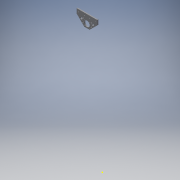
# Autodesk Inventor part: Rear Z Motor Mount
Saved by Autodesk Inventor 2017 (Build 210142000, 142)
## iProperties
Created: 2016-07-25
Part Number: Rear Z Motor Mount
Material: Generic
Document SubType Name: Modeling
Designer: User
Density: 1 g/cm^3
Appearance: Default
Author: User
Autodesk Inventor part; units mm, degrees
ref_plane "YZ Plane" through (0, 0, 0) normal (1, 0, 0) x (0, 1, 0)
ref_plane "XZ Plane" through (0, 0, 0) normal (0, 1, 0) x (-1, 0, 0)
ref_plane "XY Plane" through (0, 0, 0) normal (0, 0, 1) x (1, 0, 0)
sketch "Sketch1" plane through (0, 0, 0) normal (0, 1, 0) x (-1, 0, 0)
  line L0 (139.3953, 734.0843) -> (139.1453, 734.7093)
  line L1 (139.1453, 734.7093) -> (138.7453, 735.2093)
  line L2 (138.7453, 735.2093) -> (138.2203, 735.6093)
  line L3 (138.2203, 735.6093) -> (137.6203, 735.8593)
  line L4 (137.6203, 735.8593) -> (136.9703, 735.9593)
  line L5 (136.9703, 735.9593) -> (136.3203, 735.8593)
  line L6 (136.3203, 735.8593) -> (135.7203, 735.6093)
  line L7 (135.7203, 735.6093) -> (135.1953, 735.2093)
  line L8 (135.1953, 735.2093) -> (134.7953, 734.7093)
  line L9 (134.7953, 734.7093) -> (134.5453, 734.0843)
  line L10 (134.5453, 734.0843) -> (134.4703, 733.4343)
  line L11 (134.4703, 733.4343) -> (134.5454, 732.7843)
  line L12 (134.5454, 732.7843) -> (134.7954, 732.1844)
  line L13 (134.7954, 732.1844) -> (135.1954, 731.6593)
  line L14 (135.1954, 731.6593) -> (135.7204, 731.2593)
  line L15 (135.7204, 731.2593) -> (136.3203, 731.0093)
  line L16 (136.3203, 731.0093) -> (136.9704, 730.9343)
  line L17 (136.9704, 730.9343) -> (137.6204, 731.0094)
  line L18 (137.6204, 731.0094) -> (138.2204, 731.2594)
  line L19 (138.2204, 731.2594) -> (138.7453, 731.6593)
  line L20 (138.7453, 731.6593) -> (139.1453, 732.1843)
  line L21 (139.1453, 732.1843) -> (139.3953, 732.7843)
  line L22 (139.3953, 732.7843) -> (139.4953, 733.4341)
  line L23 (139.4953, 733.4341) -> (139.3953, 734.0843)
  line L24 (109.1446, 718.8093) -> (109.146, 712.6093)
  line L25 (109.146, 712.6093) -> (115.546, 712.6107)
  line L26 (115.546, 712.6107) -> (115.5446, 718.8107)
  line L27 (115.5446, 718.8107) -> (109.1446, 718.8093)
  line L28 (105.1702, 713.5342) -> (105.0202, 713.9092)
  line L29 (105.0202, 713.9092) -> (104.7703, 714.2342)
  line L30 (104.7703, 714.2342) -> (104.4453, 714.4842)
  line L31 (104.4453, 714.4842) -> (104.0453, 714.6593)
  line L32 (104.0453, 714.6593) -> (103.6453, 714.7093)
  line L33 (103.6453, 714.7093) -> (103.2453, 714.6593)
  line L34 (103.2453, 714.6593) -> (102.8453, 714.4842)
  line L35 (102.8453, 714.4842) -> (102.5203, 714.2343)
  line L36 (102.5203, 714.2343) -> (102.2703, 713.9093)
  line L37 (102.2703, 713.9093) -> (102.1203, 713.5343)
  line L38 (102.1203, 713.5343) -> (102.0703, 713.1093)
  line L39 (102.0703, 713.1093) -> (102.1203, 712.7093)
  line L40 (102.1203, 712.7093) -> (102.2703, 712.3093)
  line L41 (102.2703, 712.3093) -> (102.5203, 711.9843)
  line L42 (102.5203, 711.9843) -> (102.8452, 711.7343)
  line L43 (102.8452, 711.7343) -> (103.2452, 711.5841)
  line L44 (103.2452, 711.5841) -> (103.6452, 711.5341)
  line L45 (103.6452, 711.5341) -> (104.0452, 711.5841)
  line L46 (104.0452, 711.5841) -> (104.4452, 711.7341)
  line L47 (104.4452, 711.7341) -> (104.7702, 711.9841)
  line L48 (104.7702, 711.9841) -> (105.0202, 712.3091)
  line L49 (105.0202, 712.3091) -> (105.1704, 712.709)
  line L50 (105.1704, 712.709) -> (105.2452, 713.1084)
  line L51 (105.2452, 713.1084) -> (105.1702, 713.5342)
  line L52 (103.5953, 701.7594) -> (101.9953, 705.6094)
  line L53 (101.9953, 705.6094) -> (99.4703, 708.9344)
  line L54 (99.4703, 708.9344) -> (96.1453, 711.4844)
  line L55 (96.1453, 711.4844) -> (92.2953, 713.0594)
  line L56 (92.2953, 713.0594) -> (88.1453, 713.6093)
  line L57 (88.1453, 713.6093) -> (83.9953, 713.0593)
  line L58 (83.9953, 713.0593) -> (80.1453, 711.4843)
  line L59 (80.1453, 711.4843) -> (76.8203, 708.9343)
  line L60 (76.8203, 708.9343) -> (74.2953, 705.6093)
  line L61 (74.2953, 705.6093) -> (72.6953, 701.7593)
  line L62 (72.6953, 701.7593) -> (72.1453, 697.6093)
  line L63 (72.1453, 697.6093) -> (72.6953, 693.4843)
  line L64 (72.6953, 693.4843) -> (74.2953, 689.6093)
  line L65 (74.2953, 689.6093) -> (76.8203, 686.3093)
  line L66 (76.8203, 686.3093) -> (80.1453, 683.7593)
  line L67 (80.1453, 683.7593) -> (83.9953, 682.1593)
  line L68 (83.9953, 682.1593) -> (88.1453, 681.6093)
  line L69 (88.1453, 681.6093) -> (92.2953, 682.1593)
  line L70 (92.2953, 682.1593) -> (96.1453, 683.7593)
  line L71 (96.1453, 683.7593) -> (99.4703, 686.3093)
  line L72 (99.4703, 686.3093) -> (101.9953, 689.6093)
  line L73 (101.9953, 689.6093) -> (103.5953, 693.4843)
  line L74 (103.5953, 693.4843) -> (104.1453, 697.6092)
  line L75 (104.1453, 697.6092) -> (103.5953, 701.7594)
  line L76 (113.8952, 705.5088) -> (113.7453, 705.8839)
  line L77 (113.7453, 705.8839) -> (113.5201, 706.2093)
  line L78 (113.5201, 706.2093) -> (113.1952, 706.4594)
  line L79 (113.1952, 706.4594) -> (112.8451, 706.6343)
  line L80 (112.8451, 706.6343) -> (112.4451, 706.7093)
  line L81 (112.4451, 706.7093) -> (112.0451, 706.6843)
  line L82 (112.0451, 706.6843) -> (111.6701, 706.5593)
  line L83 (111.6701, 706.5593) -> (111.3201, 706.3594)
  line L84 (111.3201, 706.3594) -> (111.0451, 706.0594)
  line L85 (111.0451, 706.0594) -> (110.8702, 705.7093)
  line L86 (110.8702, 705.7093) -> (110.7703, 705.3093)
  line L87 (110.7703, 705.3093) -> (110.7703, 704.9093)
  line L88 (110.7703, 704.9093) -> (110.8704, 704.5343)
  line L89 (110.8704, 704.5343) -> (111.0454, 704.1843)
  line L90 (111.0454, 704.1843) -> (111.3203, 703.8843)
  line L91 (111.3203, 703.8843) -> (111.6703, 703.6592)
  line L92 (111.6703, 703.6592) -> (112.0453, 703.5342)
  line L93 (112.0453, 703.5342) -> (112.4453, 703.5091)
  line L94 (112.4453, 703.5091) -> (112.8453, 703.5841)
  line L95 (112.8453, 703.5841) -> (113.1954, 703.759)
  line L96 (113.1954, 703.759) -> (113.5203, 704.009)
  line L97 (113.5203, 704.009) -> (113.7452, 704.3338)
  line L98 (113.7452, 704.3338) -> (113.8952, 704.7088)
  line L99 (113.8952, 704.7088) -> (113.9453, 705.1088)
  line L100 (113.9453, 705.1088) -> (113.8952, 705.5088)
  line L101 (109.1446, 697.6093) -> (109.146, 691.4093)
  line L102 (109.146, 691.4093) -> (115.546, 691.4107)
  line L103 (115.546, 691.4107) -> (115.5446, 697.6107)
  line L104 (115.5446, 697.6107) -> (109.1446, 697.6093)
  line L105 (105.1678, 682.534) -> (105.0178, 682.909)
  line L106 (105.0178, 682.909) -> (104.7679, 683.234)
  line L107 (104.7679, 683.234) -> (104.4429, 683.484)
  line L108 (104.4429, 683.484) -> (104.0429, 683.6591)
  line L109 (104.0429, 683.6591) -> (103.6428, 683.7091)
  line L110 (103.6428, 683.7091) -> (103.2428, 683.6591)
  line L111 (103.2428, 683.6591) -> (102.8429, 683.4841)
  line L112 (102.8429, 683.4841) -> (102.5178, 683.2341)
  line L113 (102.5178, 683.2341) -> (102.2678, 682.9091)
  line L114 (102.2678, 682.9091) -> (102.1178, 682.5342)
  line L115 (102.1178, 682.5342) -> (102.0427, 682.1087)
  line L116 (102.0427, 682.1087) -> (102.1177, 681.7088)
  line L117 (102.1177, 681.7088) -> (102.2676, 681.3088)
  line L118 (102.2676, 681.3088) -> (102.5176, 680.9838)
  line L119 (102.5176, 680.9838) -> (102.8426, 680.7337)
  line L120 (102.8426, 680.7337) -> (103.2426, 680.5836)
  line L121 (103.2426, 680.5836) -> (103.6425, 680.5336)
  line L122 (103.6425, 680.5336) -> (104.0426, 680.5836)
  line L123 (104.0426, 680.5836) -> (104.4425, 680.7336)
  line L124 (104.4425, 680.7336) -> (104.7676, 680.9836)
  line L125 (104.7676, 680.9836) -> (105.0176, 681.3086)
  line L126 (105.0176, 681.3086) -> (105.1678, 681.7085)
  line L127 (105.1678, 681.7085) -> (105.2428, 682.1086)
  line L128 (105.2428, 682.1086) -> (105.1678, 682.534)
  line L129 (74.171, 682.5344) -> (74.021, 682.9094)
  line L130 (74.021, 682.9094) -> (73.7711, 683.2344)
  line L131 (73.7711, 683.2344) -> (73.4461, 683.4845)
  line L132 (73.4461, 683.4845) -> (73.0461, 683.6595)
  line L133 (73.0461, 683.6595) -> (72.6461, 683.7096)
  line L134 (72.6461, 683.7096) -> (72.2461, 683.6595)
  line L135 (72.2461, 683.6595) -> (71.8461, 683.4845)
  line L136 (71.8461, 683.4845) -> (71.5211, 683.2345)
  line L137 (71.5211, 683.2345) -> (71.2711, 682.9096)
  line L138 (71.2711, 682.9096) -> (71.1211, 682.5346)
  line L139 (71.1211, 682.5346) -> (71.0461, 682.1095)
  line L140 (71.0461, 682.1095) -> (71.121, 681.7094)
  line L141 (71.121, 681.7094) -> (71.271, 681.3095)
  line L142 (71.271, 681.3095) -> (71.521, 680.9844)
  line L143 (71.521, 680.9844) -> (71.846, 680.7344)
  line L144 (71.846, 680.7344) -> (72.2459, 680.5842)
  line L145 (72.2459, 680.5842) -> (72.6459, 680.5342)
  line L146 (72.6459, 680.5342) -> (73.0458, 680.5842)
  line L147 (73.0458, 680.5842) -> (73.4459, 680.7342)
  line L148 (73.4459, 680.7342) -> (73.7709, 680.9842)
  line L149 (73.7709, 680.9842) -> (74.0209, 681.3092)
  line L150 (74.0209, 681.3092) -> (74.1711, 681.7091)
  line L151 (74.1711, 681.7091) -> (74.246, 682.1089)
  line L152 (74.246, 682.1089) -> (74.171, 682.5344)
  line L153 (60.7446, 697.6093) -> (60.746, 691.4093)
  line L154 (60.746, 691.4093) -> (67.1456, 691.4107)
  line L155 (67.1456, 691.4107) -> (67.1442, 697.6107)
  line L156 (67.1442, 697.6107) -> (60.7446, 697.6093)
  line L157 (65.4452, 705.7089) -> (65.2453, 706.059)
  line L158 (65.2453, 706.059) -> (64.9703, 706.359)
  line L159 (64.9703, 706.359) -> (64.6204, 706.559)
  line L160 (64.6204, 706.559) -> (64.2454, 706.6841)
  line L161 (64.2454, 706.6841) -> (63.8454, 706.7092)
  line L162 (63.8454, 706.7092) -> (63.4453, 706.6342)
  line L163 (63.4453, 706.6342) -> (63.0953, 706.4592)
  line L164 (63.0953, 706.4592) -> (62.7703, 706.2093)
  line L165 (62.7703, 706.2093) -> (62.5453, 705.8843)
  line L166 (62.5453, 705.8843) -> (62.3953, 705.5093)
  line L167 (62.3953, 705.5093) -> (62.3453, 705.1093)
  line L168 (62.3453, 705.1093) -> (62.3953, 704.7093)
  line L169 (62.3953, 704.7093) -> (62.5453, 704.3343)
  line L170 (62.5453, 704.3343) -> (62.7702, 704.0093)
  line L171 (62.7702, 704.0093) -> (63.0952, 703.7592)
  line L172 (63.0952, 703.7592) -> (63.4452, 703.5842)
  line L173 (63.4452, 703.5842) -> (63.8452, 703.5092)
  line L174 (63.8452, 703.5092) -> (64.2452, 703.5342)
  line L175 (64.2452, 703.5342) -> (64.6202, 703.6591)
  line L176 (64.6202, 703.6591) -> (64.9702, 703.8841)
  line L177 (64.9702, 703.8841) -> (65.2452, 704.1841)
  line L178 (65.2452, 704.1841) -> (65.4452, 704.5341)
  line L179 (65.4452, 704.5341) -> (65.5452, 704.9091)
  line L180 (65.5452, 704.9091) -> (65.5452, 705.3089)
  line L181 (65.5452, 705.3089) -> (65.4452, 705.7089)
  line L182 (60.7203, 711.3594) -> (60.1203, 712.8093)
  line L183 (60.1203, 712.8093) -> (59.1703, 714.0343)
  line L184 (59.1703, 714.0343) -> (57.9203, 714.9843)
  line L185 (57.9203, 714.9843) -> (56.4703, 715.5843)
  line L186 (56.4703, 715.5843) -> (54.9203, 715.8093)
  line L187 (54.9203, 715.8093) -> (53.3703, 715.5843)
  line L188 (53.3703, 715.5843) -> (51.9203, 714.9843)
  line L189 (51.9203, 714.9843) -> (50.6953, 714.0343)
  line L190 (50.6953, 714.0343) -> (49.7203, 712.8093)
  line L191 (49.7203, 712.8093) -> (49.1203, 711.3593)
  line L192 (49.1203, 711.3593) -> (48.9203, 709.8093)
  line L193 (48.9203, 709.8093) -> (49.1203, 708.2343)
  line L194 (49.1203, 708.2343) -> (49.7203, 706.8093)
  line L195 (49.7203, 706.8093) -> (50.6953, 705.5593)
  line L196 (50.6953, 705.5593) -> (51.9203, 704.6093)
  line L197 (51.9203, 704.6093) -> (53.3703, 704.0093)
  line L198 (53.3703, 704.0093) -> (54.9203, 703.8093)
  line L199 (54.9203, 703.8093) -> (56.4703, 704.0093)
  line L200 (56.4703, 704.0093) -> (57.9202, 704.6093)
  line L201 (57.9202, 704.6093) -> (59.1702, 705.5594)
  line L202 (59.1702, 705.5594) -> (60.1202, 706.8094)
  line L203 (60.1202, 706.8094) -> (60.7201, 708.2344)
  line L204 (60.7201, 708.2344) -> (60.9203, 709.8095)
  line L205 (60.9203, 709.8095) -> (60.7203, 711.3594)
  line L206 (60.7446, 718.8093) -> (60.746, 712.6093)
  line L207 (60.746, 712.6093) -> (67.146, 712.6107)
  line L208 (67.146, 712.6107) -> (67.1446, 718.8107)
  line L209 (67.1446, 718.8107) -> (60.7446, 718.8093)
  line L210 (74.1702, 713.5342) -> (74.0203, 713.9092)
  line L211 (74.0203, 713.9092) -> (73.7703, 714.2342)
  line L212 (73.7703, 714.2342) -> (73.4453, 714.4842)
  line L213 (73.4453, 714.4842) -> (73.0453, 714.6593)
  line L214 (73.0453, 714.6593) -> (72.6454, 714.7093)
  line L215 (72.6454, 714.7093) -> (72.2454, 714.6593)
  line L216 (72.2454, 714.6593) -> (71.8454, 714.4843)
  line L217 (71.8454, 714.4843) -> (71.5204, 714.2343)
  line L218 (71.5204, 714.2343) -> (71.2703, 713.9093)
  line L219 (71.2703, 713.9093) -> (71.1203, 713.5343)
  line L220 (71.1203, 713.5343) -> (71.0703, 713.1093)
  line L221 (71.0703, 713.1093) -> (71.1203, 712.7093)
  line L222 (71.1203, 712.7093) -> (71.2703, 712.3093)
  line L223 (71.2703, 712.3093) -> (71.5203, 711.9843)
  line L224 (71.5203, 711.9843) -> (71.8452, 711.7342)
  line L225 (71.8452, 711.7342) -> (72.2452, 711.5841)
  line L226 (72.2452, 711.5841) -> (72.6452, 711.5341)
  line L227 (72.6452, 711.5341) -> (73.0452, 711.5841)
  line L228 (73.0452, 711.5841) -> (73.4452, 711.7341)
  line L229 (73.4452, 711.7341) -> (73.7702, 711.9841)
  line L230 (73.7702, 711.9841) -> (74.0203, 712.3091)
  line L231 (74.0203, 712.3091) -> (74.1704, 712.709)
  line L232 (74.1704, 712.709) -> (74.2453, 713.1084)
  line L233 (74.2453, 713.1084) -> (74.1702, 713.5342)
  line L234 (76.5953, 734.0843) -> (76.3453, 734.7093)
  line L235 (76.3453, 734.7093) -> (75.9453, 735.2093)
  line L236 (75.9453, 735.2093) -> (75.4203, 735.6093)
  line L237 (75.4203, 735.6093) -> (74.8203, 735.8593)
  line L238 (74.8203, 735.8593) -> (74.1703, 735.9593)
  line L239 (74.1703, 735.9593) -> (73.5203, 735.8593)
  line L240 (73.5203, 735.8593) -> (72.9203, 735.6093)
  line L241 (72.9203, 735.6093) -> (72.3953, 735.2093)
  line L242 (72.3953, 735.2093) -> (71.9953, 734.7093)
  line L243 (71.9953, 734.7093) -> (71.7453, 734.0843)
  line L244 (71.7453, 734.0843) -> (71.6703, 733.4343)
  line L245 (71.6703, 733.4343) -> (71.7453, 732.7843)
  line L246 (71.7453, 732.7843) -> (71.9954, 732.1843)
  line L247 (71.9954, 732.1843) -> (72.3953, 731.6593)
  line L248 (72.3953, 731.6593) -> (72.9203, 731.2593)
  line L249 (72.9203, 731.2593) -> (73.5203, 731.0093)
  line L250 (73.5203, 731.0093) -> (74.1704, 730.9343)
  line L251 (74.1704, 730.9343) -> (74.8203, 731.0094)
  line L252 (74.8203, 731.0094) -> (75.4203, 731.2594)
  line L253 (75.4203, 731.2594) -> (75.9453, 731.6593)
  line L254 (75.9453, 731.6593) -> (76.3453, 732.1844)
  line L255 (76.3453, 732.1844) -> (76.5953, 732.7843)
  line L256 (76.5953, 732.7843) -> (76.6953, 733.4342)
  line L257 (76.6953, 733.4342) -> (76.5953, 734.0843)
  line L258 (104.5702, 734.0842) -> (104.3202, 734.7093)
  line L259 (104.3202, 734.7093) -> (103.9202, 735.2092)
  line L260 (103.9202, 735.2092) -> (103.3952, 735.6092)
  line L261 (103.3952, 735.6092) -> (102.7703, 735.8592)
  line L262 (102.7703, 735.8592) -> (102.1203, 735.9592)
  line L263 (102.1203, 735.9592) -> (101.4702, 735.8592)
  line L264 (101.4702, 735.8592) -> (100.8452, 735.6093)
  line L265 (100.8452, 735.6093) -> (100.3202, 735.2093)
  line L266 (100.3202, 735.2093) -> (99.9202, 734.7093)
  line L267 (99.9202, 734.7093) -> (99.6702, 734.0843)
  line L268 (99.6702, 734.0843) -> (99.5702, 733.4343)
  line L269 (99.5702, 733.4343) -> (99.6702, 732.7843)
  line L270 (99.6702, 732.7843) -> (99.9202, 732.1843)
  line L271 (99.9202, 732.1843) -> (100.3202, 731.6593)
  line L272 (100.3202, 731.6593) -> (100.8452, 731.2593)
  line L273 (100.8452, 731.2593) -> (101.4702, 731.0093)
  line L274 (101.4702, 731.0093) -> (102.1202, 730.9343)
  line L275 (102.1202, 730.9343) -> (102.7702, 731.0093)
  line L276 (102.7702, 731.0093) -> (103.3952, 731.2593)
  line L277 (103.3952, 731.2593) -> (103.9201, 731.6592)
  line L278 (103.9201, 731.6592) -> (104.3201, 732.1842)
  line L279 (104.3201, 732.1842) -> (104.5701, 732.7841)
  line L280 (104.5701, 732.7841) -> (104.6702, 733.4343)
  line L281 (104.6702, 733.4343) -> (104.5702, 734.0842)
  line L282 (41.7452, 734.0843) -> (41.4953, 734.7094)
  line L283 (41.4953, 734.7094) -> (41.0953, 735.2093)
  line L284 (41.0953, 735.2093) -> (40.5703, 735.6093)
  line L285 (40.5703, 735.6093) -> (39.9703, 735.8593)
  line L286 (39.9703, 735.8593) -> (39.3203, 735.9593)
  line L287 (39.3203, 735.9593) -> (38.6703, 735.8593)
  line L288 (38.6703, 735.8593) -> (38.0703, 735.6093)
  line L289 (38.0703, 735.6093) -> (37.5453, 735.2093)
  line L290 (37.5453, 735.2093) -> (37.1453, 734.7093)
  line L291 (37.1453, 734.7093) -> (36.8953, 734.0843)
  line L292 (36.8953, 734.0843) -> (36.7953, 733.4343)
  line L293 (36.7953, 733.4343) -> (36.8953, 732.7843)
  line L294 (36.8953, 732.7843) -> (37.1453, 732.1843)
  line L295 (37.1453, 732.1843) -> (37.5453, 731.6593)
  line L296 (37.5453, 731.6593) -> (38.0703, 731.2593)
  line L297 (38.0703, 731.2593) -> (38.6703, 731.0093)
  line L298 (38.6703, 731.0093) -> (39.3203, 730.9343)
  line L299 (39.3203, 730.9343) -> (39.9703, 731.0094)
  line L300 (39.9703, 731.0094) -> (40.5703, 731.2594)
  line L301 (40.5703, 731.2594) -> (41.0953, 731.6594)
  line L302 (41.0953, 731.6594) -> (41.4953, 732.1844)
  line L303 (41.4953, 732.1844) -> (41.7453, 732.7844)
  line L304 (41.7453, 732.7844) -> (41.8203, 733.4343)
  line L305 (41.8203, 733.4343) -> (41.7452, 734.0843)
  line L306 (29.3173, 745.6342) -> (29.3233, 718.4343)
  line L307 (29.3233, 718.4343) -> (72.6578, 675.1188)
  line L308 (72.6578, 675.1188) -> (103.6578, 675.1256)
  line L309 (103.6578, 675.1256) -> (146.9733, 718.4601)
  line L310 (146.9733, 718.4601) -> (146.9673, 745.66)
  line L311 (146.9673, 745.66) -> (29.3173, 745.6342)
  line L312 (127.1703, 711.3593) -> (126.5703, 712.8093)
  line L313 (126.5703, 712.8093) -> (125.5952, 714.0343)
  line L314 (125.5952, 714.0343) -> (124.3702, 714.9843)
  line L315 (124.3702, 714.9843) -> (122.9202, 715.5843)
  line L316 (122.9202, 715.5843) -> (121.3702, 715.8093)
  line L317 (121.3702, 715.8093) -> (119.8202, 715.5843)
  line L318 (119.8202, 715.5843) -> (118.3703, 714.9843)
  line L319 (118.3703, 714.9843) -> (117.1203, 714.0342)
  line L320 (117.1203, 714.0342) -> (116.1703, 712.8092)
  line L321 (116.1703, 712.8092) -> (115.5703, 711.3592)
  line L322 (115.5703, 711.3592) -> (115.3703, 709.8092)
  line L323 (115.3703, 709.8092) -> (115.5703, 708.2342)
  line L324 (115.5703, 708.2342) -> (116.1703, 706.8092)
  line L325 (116.1703, 706.8092) -> (117.1204, 705.5592)
  line L326 (117.1204, 705.5592) -> (118.3704, 704.6093)
  line L327 (118.3704, 704.6093) -> (119.8204, 704.0093)
  line L328 (119.8204, 704.0093) -> (121.3704, 703.8093)
  line L329 (121.3704, 703.8093) -> (122.9204, 704.0093)
  line L330 (122.9204, 704.0093) -> (124.3704, 704.6093)
  line L331 (124.3704, 704.6093) -> (125.5954, 705.5593)
  line L332 (125.5954, 705.5593) -> (126.5701, 706.8093)
  line L333 (126.5701, 706.8093) -> (127.1701, 708.2343)
  line L334 (127.1701, 708.2343) -> (127.3703, 709.8093)
  line L335 (127.3703, 709.8093) -> (127.1703, 711.3593)
  point P0 (0, 0)
  constraints: 672 end point, 122 parallel, 97 perpendicular
extrude "Extrusion1" add sketch "Sketch1" along normal blind 6 contours L281 L280 L279 L278 L277 L276 L275 L274 L273 L272 L271 L270 L269 L268 L267 L266 L265 L264 L263 L262 L261 L260 L259 L258 | L311 L310 L309 L308 L307 L306
sketch "Sketch2" plane through (0, 0, 0) normal (0, -1, 0) x (1, 0, 0)
  line L0 (-104.1453, 697.6092) -> (-103.5953, 701.7594) projected
  line L1 (-103.5953, 701.7594) -> (-101.9953, 705.6094) projected
  line L2 (-101.9953, 705.6094) -> (-99.4703, 708.9344) projected
  line L3 (-99.4703, 708.9344) -> (-96.1453, 711.4844) projected
  line L4 (-96.1453, 711.4844) -> (-92.2953, 713.0594) projected
  line L5 (-92.2953, 713.0594) -> (-88.1453, 713.6093) projected
  line L6 (-88.1453, 713.6093) -> (-83.9953, 713.0593) projected
  line L7 (-83.9953, 713.0593) -> (-80.1453, 711.4843) projected
  line L8 (-80.1453, 711.4843) -> (-76.8203, 708.9343) projected
  line L9 (-76.8203, 708.9343) -> (-74.2953, 705.6093) projected
  line L10 (-74.2953, 705.6093) -> (-72.6953, 701.7593) projected
  line L11 (-72.6953, 701.7593) -> (-72.1453, 697.6093) projected
  line L12 (-72.1453, 697.6093) -> (-72.6953, 693.4843) projected
  line L13 (-72.6953, 693.4843) -> (-74.2953, 689.6093) projected
  line L14 (-74.2953, 689.6093) -> (-76.8203, 686.3093) projected
  line L15 (-76.8203, 686.3093) -> (-80.1453, 683.7593) projected
  line L16 (-80.1453, 683.7593) -> (-83.9953, 682.1593) projected
  line L17 (-83.9953, 682.1593) -> (-88.1453, 681.6093) projected
  line L18 (-88.1453, 681.6093) -> (-92.2953, 682.1593) projected
  line L19 (-92.2953, 682.1593) -> (-96.1453, 683.7593) projected
  line L20 (-96.1453, 683.7593) -> (-99.4703, 686.3093) projected
  line L21 (-99.4703, 686.3093) -> (-101.9953, 689.6093) projected
  line L22 (-101.9953, 689.6093) -> (-103.5953, 693.4843) projected
  line L23 (-103.5953, 693.4843) -> (-104.1453, 697.6092) projected
  line L24 (-127.3703, 709.8093) -> (-127.1703, 711.3593) projected
  line L25 (-127.1703, 711.3593) -> (-126.5703, 712.8093) projected
  line L26 (-126.5703, 712.8093) -> (-125.5952, 714.0343) projected
  line L27 (-125.5952, 714.0343) -> (-124.3702, 714.9843) projected
  line L28 (-124.3702, 714.9843) -> (-122.9202, 715.5843) projected
  line L29 (-122.9202, 715.5843) -> (-121.3702, 715.8093) projected
  line L30 (-121.3702, 715.8093) -> (-119.8202, 715.5843) projected
  line L31 (-119.8202, 715.5843) -> (-118.3703, 714.9843) projected
  line L32 (-118.3703, 714.9843) -> (-117.1203, 714.0342) projected
  line L33 (-117.1203, 714.0342) -> (-116.1703, 712.8092) projected
  line L34 (-116.1703, 712.8092) -> (-115.5703, 711.3592) projected
  line L35 (-115.5703, 711.3592) -> (-115.3703, 709.8092) projected
  line L36 (-115.3703, 709.8092) -> (-115.5703, 708.2342) projected
  line L37 (-115.5703, 708.2342) -> (-116.1703, 706.8092) projected
  line L38 (-116.1703, 706.8092) -> (-117.1204, 705.5592) projected
  line L39 (-117.1204, 705.5592) -> (-118.3704, 704.6093) projected
  line L40 (-118.3704, 704.6093) -> (-119.8204, 704.0093) projected
  line L41 (-119.8204, 704.0093) -> (-121.3704, 703.8093) projected
  line L42 (-121.3704, 703.8093) -> (-122.9204, 704.0093) projected
  line L43 (-122.9204, 704.0093) -> (-124.3704, 704.6093) projected
  line L44 (-124.3704, 704.6093) -> (-125.5954, 705.5593) projected
  line L45 (-125.5954, 705.5593) -> (-126.5701, 706.8093) projected
  line L46 (-126.5701, 706.8093) -> (-127.1701, 708.2343) projected
  line L47 (-127.1701, 708.2343) -> (-127.3703, 709.8093) projected
  line L48 (-60.9203, 709.8095) -> (-60.7203, 711.3594) projected
  line L49 (-60.7203, 711.3594) -> (-60.1203, 712.8093) projected
  line L50 (-60.1203, 712.8093) -> (-59.1703, 714.0343) projected
  line L51 (-59.1703, 714.0343) -> (-57.9203, 714.9843) projected
  line L52 (-57.9203, 714.9843) -> (-56.4703, 715.5843) projected
  line L53 (-56.4703, 715.5843) -> (-54.9203, 715.8093) projected
  line L54 (-54.9203, 715.8093) -> (-53.3703, 715.5843) projected
  line L55 (-53.3703, 715.5843) -> (-51.9203, 714.9843) projected
  line L56 (-51.9203, 714.9843) -> (-50.6953, 714.0343) projected
  line L57 (-50.6953, 714.0343) -> (-49.7203, 712.8093) projected
  line L58 (-49.7203, 712.8093) -> (-49.1203, 711.3593) projected
  line L59 (-49.1203, 711.3593) -> (-48.9203, 709.8093) projected
  line L60 (-48.9203, 709.8093) -> (-49.1203, 708.2343) projected
  line L61 (-49.1203, 708.2343) -> (-49.7203, 706.8093) projected
  line L62 (-49.7203, 706.8093) -> (-50.6953, 705.5593) projected
  line L63 (-50.6953, 705.5593) -> (-51.9203, 704.6093) projected
  line L64 (-51.9203, 704.6093) -> (-53.3703, 704.0093) projected
  line L65 (-53.3703, 704.0093) -> (-54.9203, 703.8093) projected
  line L66 (-54.9203, 703.8093) -> (-56.4703, 704.0093) projected
  line L67 (-56.4703, 704.0093) -> (-57.9202, 704.6093) projected
  line L68 (-57.9202, 704.6093) -> (-59.1702, 705.5594) projected
  line L69 (-59.1702, 705.5594) -> (-60.1202, 706.8094) projected
  line L70 (-60.1202, 706.8094) -> (-60.7201, 708.2344) projected
  line L71 (-60.7201, 708.2344) -> (-60.9203, 709.8095) projected
  line L72 (-67.1446, 718.8107) -> (-60.7446, 718.8093) projected
  line L73 (-60.7446, 718.8093) -> (-60.746, 712.6093) projected
  line L74 (-60.746, 712.6093) -> (-67.146, 712.6107) projected
  line L75 (-67.146, 712.6107) -> (-67.1446, 718.8107) projected
  line L76 (-115.5446, 697.6107) -> (-109.1446, 697.6093) projected
  line L77 (-109.1446, 697.6093) -> (-109.146, 691.4093) projected
  line L78 (-109.146, 691.4093) -> (-115.546, 691.4107) projected
  line L79 (-115.546, 691.4107) -> (-115.5446, 697.6107) projected
  line L80 (-115.5446, 718.8107) -> (-109.1446, 718.8093) projected
  line L81 (-109.1446, 718.8093) -> (-109.146, 712.6093) projected
  line L82 (-109.146, 712.6093) -> (-115.546, 712.6107) projected
  line L83 (-115.546, 712.6107) -> (-115.5446, 718.8107) projected
  line L84 (-67.1442, 697.6107) -> (-60.7446, 697.6093) projected
  line L85 (-60.7446, 697.6093) -> (-60.746, 691.4093) projected
  line L86 (-60.746, 691.4093) -> (-67.1456, 691.4107) projected
  line L87 (-67.1456, 691.4107) -> (-67.1442, 697.6107) projected
  line L88 (-139.4953, 733.4341) -> (-139.3953, 734.0843) projected
  line L89 (-139.3953, 734.0843) -> (-139.1453, 734.7093) projected
  line L90 (-139.1453, 734.7093) -> (-138.7453, 735.2093) projected
  line L91 (-138.7453, 735.2093) -> (-138.2203, 735.6093) projected
  line L92 (-138.2203, 735.6093) -> (-137.6203, 735.8593) projected
  line L93 (-137.6203, 735.8593) -> (-136.9703, 735.9593) projected
  line L94 (-136.9703, 735.9593) -> (-136.3203, 735.8593) projected
  line L95 (-136.3203, 735.8593) -> (-135.7203, 735.6093) projected
  line L96 (-135.7203, 735.6093) -> (-135.1953, 735.2093) projected
  line L97 (-135.1953, 735.2093) -> (-134.7953, 734.7093) projected
  line L98 (-134.7953, 734.7093) -> (-134.5453, 734.0843) projected
  line L99 (-134.5453, 734.0843) -> (-134.4703, 733.4343) projected
  line L100 (-134.4703, 733.4343) -> (-134.5454, 732.7843) projected
  line L101 (-134.5454, 732.7843) -> (-134.7954, 732.1844) projected
  line L102 (-134.7954, 732.1844) -> (-135.1954, 731.6593) projected
  line L103 (-135.1954, 731.6593) -> (-135.7204, 731.2593) projected
  line L104 (-135.7204, 731.2593) -> (-136.3203, 731.0093) projected
  line L105 (-136.3203, 731.0093) -> (-136.9704, 730.9343) projected
  line L106 (-136.9704, 730.9343) -> (-137.6204, 731.0094) projected
  line L107 (-137.6204, 731.0094) -> (-138.2204, 731.2594) projected
  line L108 (-138.2204, 731.2594) -> (-138.7453, 731.6593) projected
  line L109 (-138.7453, 731.6593) -> (-139.1453, 732.1843) projected
  line L110 (-139.1453, 732.1843) -> (-139.3953, 732.7843) projected
  line L111 (-139.3953, 732.7843) -> (-139.4953, 733.4341) projected
  line L112 (-41.8203, 733.4343) -> (-41.7452, 734.0843) projected
  line L113 (-41.7452, 734.0843) -> (-41.4953, 734.7094) projected
  line L114 (-41.4953, 734.7094) -> (-41.0953, 735.2093) projected
  line L115 (-41.0953, 735.2093) -> (-40.5703, 735.6093) projected
  line L116 (-40.5703, 735.6093) -> (-39.9703, 735.8593) projected
  line L117 (-39.9703, 735.8593) -> (-39.3203, 735.9593) projected
  line L118 (-39.3203, 735.9593) -> (-38.6703, 735.8593) projected
  line L119 (-38.6703, 735.8593) -> (-38.0703, 735.6093) projected
  line L120 (-38.0703, 735.6093) -> (-37.5453, 735.2093) projected
  line L121 (-37.5453, 735.2093) -> (-37.1453, 734.7093) projected
  line L122 (-37.1453, 734.7093) -> (-36.8953, 734.0843) projected
  line L123 (-36.8953, 734.0843) -> (-36.7953, 733.4343) projected
  line L124 (-36.7953, 733.4343) -> (-36.8953, 732.7843) projected
  line L125 (-36.8953, 732.7843) -> (-37.1453, 732.1843) projected
  line L126 (-37.1453, 732.1843) -> (-37.5453, 731.6593) projected
  line L127 (-37.5453, 731.6593) -> (-38.0703, 731.2593) projected
  line L128 (-38.0703, 731.2593) -> (-38.6703, 731.0093) projected
  line L129 (-38.6703, 731.0093) -> (-39.3203, 730.9343) projected
  line L130 (-39.3203, 730.9343) -> (-39.9703, 731.0094) projected
  line L131 (-39.9703, 731.0094) -> (-40.5703, 731.2594) projected
  line L132 (-40.5703, 731.2594) -> (-41.0953, 731.6594) projected
  line L133 (-41.0953, 731.6594) -> (-41.4953, 732.1844) projected
  line L134 (-41.4953, 732.1844) -> (-41.7453, 732.7844) projected
  line L135 (-41.7453, 732.7844) -> (-41.8203, 733.4343) projected
  line L136 (-76.6953, 733.4342) -> (-76.5953, 734.0843) projected
  line L137 (-76.5953, 734.0843) -> (-76.3453, 734.7093) projected
  line L138 (-76.3453, 734.7093) -> (-75.9453, 735.2093) projected
  line L139 (-75.9453, 735.2093) -> (-75.4203, 735.6093) projected
  line L140 (-75.4203, 735.6093) -> (-74.8203, 735.8593) projected
  line L141 (-74.8203, 735.8593) -> (-74.1703, 735.9593) projected
  line L142 (-74.1703, 735.9593) -> (-73.5203, 735.8593) projected
  line L143 (-73.5203, 735.8593) -> (-72.9203, 735.6093) projected
  line L144 (-72.9203, 735.6093) -> (-72.3953, 735.2093) projected
  line L145 (-72.3953, 735.2093) -> (-71.9953, 734.7093) projected
  line L146 (-71.9953, 734.7093) -> (-71.7453, 734.0843) projected
  line L147 (-71.7453, 734.0843) -> (-71.6703, 733.4343) projected
  line L148 (-71.6703, 733.4343) -> (-71.7453, 732.7843) projected
  line L149 (-71.7453, 732.7843) -> (-71.9954, 732.1843) projected
  line L150 (-71.9954, 732.1843) -> (-72.3953, 731.6593) projected
  line L151 (-72.3953, 731.6593) -> (-72.9203, 731.2593) projected
  line L152 (-72.9203, 731.2593) -> (-73.5203, 731.0093) projected
  line L153 (-73.5203, 731.0093) -> (-74.1704, 730.9343) projected
  line L154 (-74.1704, 730.9343) -> (-74.8203, 731.0094) projected
  line L155 (-74.8203, 731.0094) -> (-75.4203, 731.2594) projected
  line L156 (-75.4203, 731.2594) -> (-75.9453, 731.6593) projected
  line L157 (-75.9453, 731.6593) -> (-76.3453, 732.1844) projected
  line L158 (-76.3453, 732.1844) -> (-76.5953, 732.7843) projected
  line L159 (-76.5953, 732.7843) -> (-76.6953, 733.4342) projected
  line L160 (-65.5452, 705.3089) -> (-65.4452, 705.7089) projected
  line L161 (-65.4452, 705.7089) -> (-65.2453, 706.059) projected
  line L162 (-65.2453, 706.059) -> (-64.9703, 706.359) projected
  line L163 (-64.9703, 706.359) -> (-64.6204, 706.559) projected
  line L164 (-64.6204, 706.559) -> (-64.2454, 706.6841) projected
  line L165 (-64.2454, 706.6841) -> (-63.8454, 706.7092) projected
  line L166 (-63.8454, 706.7092) -> (-63.4453, 706.6342) projected
  line L167 (-63.4453, 706.6342) -> (-63.0953, 706.4592) projected
  line L168 (-63.0953, 706.4592) -> (-62.7703, 706.2093) projected
  line L169 (-62.7703, 706.2093) -> (-62.5453, 705.8843) projected
  line L170 (-62.5453, 705.8843) -> (-62.3953, 705.5093) projected
  line L171 (-62.3953, 705.5093) -> (-62.3453, 705.1093) projected
  line L172 (-62.3453, 705.1093) -> (-62.3953, 704.7093) projected
  line L173 (-62.3953, 704.7093) -> (-62.5453, 704.3343) projected
  line L174 (-62.5453, 704.3343) -> (-62.7702, 704.0093) projected
  line L175 (-62.7702, 704.0093) -> (-63.0952, 703.7592) projected
  line L176 (-63.0952, 703.7592) -> (-63.4452, 703.5842) projected
  line L177 (-63.4452, 703.5842) -> (-63.8452, 703.5092) projected
  line L178 (-63.8452, 703.5092) -> (-64.2452, 703.5342) projected
  line L179 (-64.2452, 703.5342) -> (-64.6202, 703.6591) projected
  line L180 (-64.6202, 703.6591) -> (-64.9702, 703.8841) projected
  line L181 (-64.9702, 703.8841) -> (-65.2452, 704.1841) projected
  line L182 (-65.2452, 704.1841) -> (-65.4452, 704.5341) projected
  line L183 (-65.4452, 704.5341) -> (-65.5452, 704.9091) projected
  line L184 (-65.5452, 704.9091) -> (-65.5452, 705.3089) projected
  line L185 (-113.9453, 705.1088) -> (-113.8952, 705.5088) projected
  line L186 (-113.8952, 705.5088) -> (-113.7453, 705.8839) projected
  line L187 (-113.7453, 705.8839) -> (-113.5201, 706.2093) projected
  line L188 (-113.5201, 706.2093) -> (-113.1952, 706.4594) projected
  line L189 (-113.1952, 706.4594) -> (-112.8451, 706.6343) projected
  line L190 (-112.8451, 706.6343) -> (-112.4451, 706.7093) projected
  line L191 (-112.4451, 706.7093) -> (-112.0451, 706.6843) projected
  line L192 (-112.0451, 706.6843) -> (-111.6701, 706.5593) projected
  line L193 (-111.6701, 706.5593) -> (-111.3201, 706.3594) projected
  line L194 (-111.3201, 706.3594) -> (-111.0451, 706.0594) projected
  line L195 (-111.0451, 706.0594) -> (-110.8702, 705.7093) projected
  line L196 (-110.8702, 705.7093) -> (-110.7703, 705.3093) projected
  line L197 (-110.7703, 705.3093) -> (-110.7703, 704.9093) projected
  line L198 (-110.7703, 704.9093) -> (-110.8704, 704.5343) projected
  line L199 (-110.8704, 704.5343) -> (-111.0454, 704.1843) projected
  line L200 (-111.0454, 704.1843) -> (-111.3203, 703.8843) projected
  line L201 (-111.3203, 703.8843) -> (-111.6703, 703.6592) projected
  line L202 (-111.6703, 703.6592) -> (-112.0453, 703.5342) projected
  line L203 (-112.0453, 703.5342) -> (-112.4453, 703.5091) projected
  line L204 (-112.4453, 703.5091) -> (-112.8453, 703.5841) projected
  line L205 (-112.8453, 703.5841) -> (-113.1954, 703.759) projected
  line L206 (-113.1954, 703.759) -> (-113.5203, 704.009) projected
  line L207 (-113.5203, 704.009) -> (-113.7452, 704.3338) projected
  line L208 (-113.7452, 704.3338) -> (-113.8952, 704.7088) projected
  line L209 (-113.8952, 704.7088) -> (-113.9453, 705.1088) projected
  line L210 (-105.2428, 682.1086) -> (-105.1678, 682.534) projected
  line L211 (-105.1678, 682.534) -> (-105.0178, 682.909) projected
  line L212 (-105.0178, 682.909) -> (-104.7679, 683.234) projected
  line L213 (-104.7679, 683.234) -> (-104.4429, 683.484) projected
  line L214 (-104.4429, 683.484) -> (-104.0429, 683.6591) projected
  line L215 (-104.0429, 683.6591) -> (-103.6428, 683.7091) projected
  line L216 (-103.6428, 683.7091) -> (-103.2428, 683.6591) projected
  line L217 (-103.2428, 683.6591) -> (-102.8429, 683.4841) projected
  line L218 (-102.8429, 683.4841) -> (-102.5178, 683.2341) projected
  line L219 (-102.5178, 683.2341) -> (-102.2678, 682.9091) projected
  line L220 (-102.2678, 682.9091) -> (-102.1178, 682.5342) projected
  line L221 (-102.1178, 682.5342) -> (-102.0427, 682.1087) projected
  line L222 (-102.0427, 682.1087) -> (-102.1177, 681.7088) projected
  line L223 (-102.1177, 681.7088) -> (-102.2676, 681.3088) projected
  line L224 (-102.2676, 681.3088) -> (-102.5176, 680.9838) projected
  line L225 (-102.5176, 680.9838) -> (-102.8426, 680.7337) projected
  line L226 (-102.8426, 680.7337) -> (-103.2426, 680.5836) projected
  line L227 (-103.2426, 680.5836) -> (-103.6425, 680.5336) projected
  line L228 (-103.6425, 680.5336) -> (-104.0426, 680.5836) projected
  line L229 (-104.0426, 680.5836) -> (-104.4425, 680.7336) projected
  line L230 (-104.4425, 680.7336) -> (-104.7676, 680.9836) projected
  line L231 (-104.7676, 680.9836) -> (-105.0176, 681.3086) projected
  line L232 (-105.0176, 681.3086) -> (-105.1678, 681.7085) projected
  line L233 (-105.1678, 681.7085) -> (-105.2428, 682.1086) projected
  line L234 (-74.246, 682.1089) -> (-74.171, 682.5344) projected
  line L235 (-74.171, 682.5344) -> (-74.021, 682.9094) projected
  line L236 (-74.021, 682.9094) -> (-73.7711, 683.2344) projected
  line L237 (-73.7711, 683.2344) -> (-73.4461, 683.4845) projected
  line L238 (-73.4461, 683.4845) -> (-73.0461, 683.6595) projected
  line L239 (-73.0461, 683.6595) -> (-72.6461, 683.7096) projected
  line L240 (-72.6461, 683.7096) -> (-72.2461, 683.6595) projected
  line L241 (-72.2461, 683.6595) -> (-71.8461, 683.4845) projected
  line L242 (-71.8461, 683.4845) -> (-71.5211, 683.2345) projected
  line L243 (-71.5211, 683.2345) -> (-71.2711, 682.9096) projected
  line L244 (-71.2711, 682.9096) -> (-71.1211, 682.5346) projected
  line L245 (-71.1211, 682.5346) -> (-71.0461, 682.1095) projected
  line L246 (-71.0461, 682.1095) -> (-71.121, 681.7094) projected
  line L247 (-71.121, 681.7094) -> (-71.271, 681.3095) projected
  line L248 (-71.271, 681.3095) -> (-71.521, 680.9844) projected
  line L249 (-71.521, 680.9844) -> (-71.846, 680.7344) projected
  line L250 (-71.846, 680.7344) -> (-72.2459, 680.5842) projected
  line L251 (-72.2459, 680.5842) -> (-72.6459, 680.5342) projected
  line L252 (-72.6459, 680.5342) -> (-73.0458, 680.5842) projected
  line L253 (-73.0458, 680.5842) -> (-73.4459, 680.7342) projected
  line L254 (-73.4459, 680.7342) -> (-73.7709, 680.9842) projected
  line L255 (-73.7709, 680.9842) -> (-74.0209, 681.3092) projected
  line L256 (-74.0209, 681.3092) -> (-74.1711, 681.7091) projected
  line L257 (-74.1711, 681.7091) -> (-74.246, 682.1089) projected
  line L258 (-74.2453, 713.1084) -> (-74.1702, 713.5342) projected
  line L259 (-74.1702, 713.5342) -> (-74.0203, 713.9092) projected
  line L260 (-74.0203, 713.9092) -> (-73.7703, 714.2342) projected
  line L261 (-73.7703, 714.2342) -> (-73.4453, 714.4842) projected
  line L262 (-73.4453, 714.4842) -> (-73.0453, 714.6593) projected
  line L263 (-73.0453, 714.6593) -> (-72.6454, 714.7093) projected
  line L264 (-72.6454, 714.7093) -> (-72.2454, 714.6593) projected
  line L265 (-72.2454, 714.6593) -> (-71.8454, 714.4843) projected
  line L266 (-71.8454, 714.4843) -> (-71.5204, 714.2343) projected
  line L267 (-71.5204, 714.2343) -> (-71.2703, 713.9093) projected
  line L268 (-71.2703, 713.9093) -> (-71.1203, 713.5343) projected
  line L269 (-71.1203, 713.5343) -> (-71.0703, 713.1093) projected
  line L270 (-71.0703, 713.1093) -> (-71.1203, 712.7093) projected
  line L271 (-71.1203, 712.7093) -> (-71.2703, 712.3093) projected
  line L272 (-71.2703, 712.3093) -> (-71.5203, 711.9843) projected
  line L273 (-71.5203, 711.9843) -> (-71.8452, 711.7342) projected
  line L274 (-71.8452, 711.7342) -> (-72.2452, 711.5841) projected
  line L275 (-72.2452, 711.5841) -> (-72.6452, 711.5341) projected
  line L276 (-72.6452, 711.5341) -> (-73.0452, 711.5841) projected
  line L277 (-73.0452, 711.5841) -> (-73.4452, 711.7341) projected
  line L278 (-73.4452, 711.7341) -> (-73.7702, 711.9841) projected
  line L279 (-73.7702, 711.9841) -> (-74.0203, 712.3091) projected
  line L280 (-74.0203, 712.3091) -> (-74.1704, 712.709) projected
  line L281 (-74.1704, 712.709) -> (-74.2453, 713.1084) projected
  line L282 (-105.2452, 713.1084) -> (-105.1702, 713.5342) projected
  line L283 (-105.1702, 713.5342) -> (-105.0202, 713.9092) projected
  line L284 (-105.0202, 713.9092) -> (-104.7703, 714.2342) projected
  line L285 (-104.7703, 714.2342) -> (-104.4453, 714.4842) projected
  line L286 (-104.4453, 714.4842) -> (-104.0453, 714.6593) projected
  line L287 (-104.0453, 714.6593) -> (-103.6453, 714.7093) projected
  line L288 (-103.6453, 714.7093) -> (-103.2453, 714.6593) projected
  line L289 (-103.2453, 714.6593) -> (-102.8453, 714.4842) projected
  line L290 (-102.8453, 714.4842) -> (-102.5203, 714.2343) projected
  line L291 (-102.5203, 714.2343) -> (-102.2703, 713.9093) projected
  line L292 (-102.2703, 713.9093) -> (-102.1203, 713.5343) projected
  line L293 (-102.1203, 713.5343) -> (-102.0703, 713.1093) projected
  line L294 (-102.0703, 713.1093) -> (-102.1203, 712.7093) projected
  line L295 (-102.1203, 712.7093) -> (-102.2703, 712.3093) projected
  line L296 (-102.2703, 712.3093) -> (-102.5203, 711.9843) projected
  line L297 (-102.5203, 711.9843) -> (-102.8452, 711.7343) projected
  line L298 (-102.8452, 711.7343) -> (-103.2452, 711.5841) projected
  line L299 (-103.2452, 711.5841) -> (-103.6452, 711.5341) projected
  line L300 (-103.6452, 711.5341) -> (-104.0452, 711.5841) projected
  line L301 (-104.0452, 711.5841) -> (-104.4452, 711.7341) projected
  line L302 (-104.4452, 711.7341) -> (-104.7702, 711.9841) projected
  line L303 (-104.7702, 711.9841) -> (-105.0202, 712.3091) projected
  line L304 (-105.0202, 712.3091) -> (-105.1704, 712.709) projected
  line L305 (-105.1704, 712.709) -> (-105.2452, 713.1084) projected
  line L306 (-29.3173, 745.6342) -> (-29.3233, 718.4343) projected
  line L307 (-146.9673, 745.66) -> (-29.3173, 745.6342) projected
  line L308 (-146.9733, 718.4601) -> (-146.9673, 745.66) projected
  line L309 (-103.6578, 675.1256) -> (-146.9733, 718.4601) projected
  line L310 (-72.6578, 675.1188) -> (-103.6578, 675.1256) projected
  line L311 (-29.3233, 718.4343) -> (-72.6578, 675.1188) projected
  line L312 (-83.9953, 713.0593) -> (-88.1453, 713.6093) projected
  circle A0 centre (-88.1453, 697.6093) radius 16
  point P0 (0, 0)
  constraints: 1 centre point
extrude "Extrusion2" cut sketch "Sketch2" against normal blind 6 contours A0 L2 L1 L0 | L0 L1 L2 A0 L3 L4 L5 L6 L7 L8 L9 L10 L11 L12 L13 L14 L15 L16 L17 L18 L19 L20 L21 L22 L23 | L23 L22 L21 A0 | L20 L19 L18 A0 | L17 L16 L15 A0 | A0 L3 | L14 L13 L12 A0 | L11 L10 L9 A0 | A0 L5 L4 | A0 L7 L6 | L8 A0
sketch "Sketch3" plane through (0, 0, 0) normal (0, -1, 0) x (1, 0, 0)
  line L0 (-122.9202, 715.5843) -> (-121.3702, 715.8093) projected
  line L1 (-121.3702, 715.8093) -> (-121.3704, 703.8093)
  circle A0 centre (-121.3703, 709.8093) radius 6
  line L2 (-56.4703, 715.5843) -> (-54.9203, 715.8093) projected
  line L3 (-53.3703, 704.0093) -> (-54.9203, 703.8093) projected
  line L4 (-54.9203, 715.8093) -> (-54.9203, 703.8093)
  circle A1 centre (-54.9203, 709.8093) radius 6
  line L5 (-112.8451, 706.6343) -> (-112.4451, 706.7093) projected
  line L6 (-112.0453, 703.5342) -> (-112.4453, 703.5091) projected
  line L7 (-112.4451, 706.7093) -> (-112.4453, 703.5091)
  line L8 (-104.0453, 714.6593) -> (-103.6453, 714.7093) projected
  line L9 (-103.2452, 711.5841) -> (-103.6452, 711.5341) projected
  line L10 (-103.6453, 714.7093) -> (-103.6452, 711.5341)
  line L11 (-73.0453, 714.6593) -> (-72.6454, 714.7093) projected
  line L12 (-72.2452, 711.5841) -> (-72.6452, 711.5341) projected
  line L13 (-72.6454, 714.7093) -> (-72.6452, 711.5341)
  line L14 (-63.8454, 706.7092) -> (-63.4453, 706.6342) projected
  line L15 (-63.8454, 706.7092) -> (-63.8454, 703.5091)
  line L16 (-104.0429, 683.6591) -> (-103.6428, 683.7091) projected
  line L17 (-103.2426, 680.5836) -> (-103.6425, 680.5336) projected
  line L18 (-103.6428, 683.7091) -> (-103.6425, 680.5336)
  line L19 (-72.2459, 680.5842) -> (-72.6459, 680.5342) projected
  line L20 (-72.6459, 683.712) -> (-72.6459, 680.5342)
  circle A2 centre (-112.4452, 705.1092) radius 1.6
  circle A3 centre (-103.6452, 713.1217) radius 1.6
  circle A4 centre (-72.6453, 713.1217) radius 1.6
  circle A5 centre (-63.8454, 705.1091) radius 1.6
  circle A6 centre (-72.6459, 682.1231) radius 1.6
  circle A7 centre (-103.6427, 682.1214) radius 1.6
  line L21 (-137.6203, 735.8593) -> (-136.9703, 735.9593) projected
  line L22 (-136.9704, 730.9343) -> (-136.3203, 731.0093) projected
  line L23 (-136.9703, 735.9593) -> (-136.9704, 730.9343)
  line L24 (-74.2459, 735.9593) -> (-74.2459, 730.9343)
  line L25 (-39.3203, 735.9593) -> (-38.6703, 735.8593) projected
  line L26 (-38.6703, 731.0093) -> (-39.3203, 730.9343) projected
  line L27 (-39.3203, 735.9593) -> (-39.3203, 730.9343)
  circle A8 centre (-136.9703, 733.4468) radius 2.6
  circle A9 centre (-74.2459, 733.4468) radius 2.6
  circle A10 centre (-39.3203, 733.4468) radius 2.6
  line L28 (-146.9673, 745.66) -> (-29.3173, 745.6342) projected
  line L29 (-88.1423, 745.6471) -> (-88.1423, 725.2997)
  circle A11 centre (-102.0388, 733.4468) radius 2.6
  point P0 (0, 0)
  dimension "d4" = 12
  dimension "d5" = 12
  dimension "d6" = 3.2
  dimension "d7" = 3.2
  dimension "d8" = 3.2
  dimension "d9" = 3.2
  dimension "d10" = 3.2
  dimension "d11" = 3.2
  dimension "d12" = 5.2
  dimension "d13" = 5.2
  dimension "d14" = 5.2
  constraints: 24 end point, 12 centre point, 12 midpoint, 4 vertical, 1 symmetric about line, 1 other
  measures "d4" diameter of A0
  measures "d5" diameter of A1
  measures "d6" diameter of A2
  measures "d7" diameter of A3
  measures "d8" diameter of A4
  measures "d9" diameter of A5
  measures "d10" diameter of A6
  measures "d11" diameter of A7
  measures "d12" diameter of A8
  measures "d13" diameter of A9
  measures "d14" diameter of A10
sketch "Sketch4" plane through (0, 0, 0) normal (0, -1, 0) x (1, 0, 0)
  point P0 (0, 0)
extrude "Extrusion3" cut sketch "Sketch3" against normal blind 6
body "Solid1"
